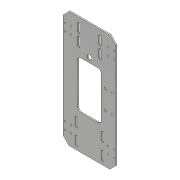
# Autodesk Inventor part: Plataina_eje_Y
Saved by Autodesk Inventor 2017 (Build 210142000, 142)
## iProperties
Created: 2018-02-17
Part Number: Plataina_eje_Y
Material: Aluminum 1100-O
Document SubType Name: Modeling
Designer: Juan Carlos Botero
Density: 2.7 g/cm^3
Appearance: Satin
Mass: 2621.1 g
Surface Area: 2107.17 cm^2
Volume: 970.778 cm^3
Author: Juan Carlos Botero
Autodesk Inventor part; units mm, degrees
ref_plane "YZ Plane" through (0, 0, 0) normal (1, 0, 0) x (0, 1, 0)
ref_plane "XZ Plane" through (0, 0, 0) normal (0, 1, 0) x (-1, 0, 0)
ref_plane "XY Plane" through (0, 0, 0) normal (0, 0, 1) x (1, 0, 0)
sketch "Sketch1" plane through (0, 0, 0) normal (0, 1, 0) x (-1, 0, 0)
  line L0 (111, 210) -> (-111, 210)
  line L1 (-111, 210) -> (-111, -210)
  line L2 (-111, -210) -> (111, -210)
  line L3 (111, -210) -> (111, 210)
  line L4 (111, 210) -> (-111, -210) construction
  line L5 (-111, 210) -> (111, -210) construction
  line L6 (111, -210) -> (75, -210) construction
  line L7 (75, -210) -> (75, -168) construction
  line L8 (75, -168) -> (111, -168) construction
  line L9 (111, -168) -> (111, -210) construction
  line L10 (-111, -210) -> (-75, -210) construction
  line L11 (-75, -210) -> (-75, -168) construction
  line L12 (-75, -168) -> (-111, -168) construction
  line L13 (-111, -168) -> (-111, -210) construction
  line L14 (-111, 210) -> (-75, 210) construction
  line L15 (-75, 210) -> (-75, 209.4774) construction
  line L16 (-75, 209.4774) -> (-111, 209.4774) construction
  line L17 (-111, 209.4774) -> (-111, 210) construction
  line L18 (111, 210) -> (75, 210) construction
  line L19 (75, 210) -> (75, 209.4774) construction
  line L20 (75, 209.4774) -> (111, 209.4774) construction
  line L21 (111, 209.4774) -> (111, 210) construction
  line L22 (75, -100) -> (-75, -100) construction
  line L23 (-75, -100) -> (-75, -210) construction
  line L24 (-75, -210) -> (75, -210) construction
  line L25 (75, -210) -> (75, -100) construction
  line L26 (75, -100) -> (-75, -210) construction
  line L27 (-75, -100) -> (75, -210) construction
  line L28 (37.5, 210) -> (-37.5, 210) construction
  line L29 (-37.5, 210) -> (-37.5, 60) construction
  line L30 (-37.5, 60) -> (37.5, 60) construction
  line L31 (37.5, 60) -> (37.5, 210) construction
  line L32 (37.5, 210) -> (-37.5, 60) construction
  line L33 (-37.5, 210) -> (37.5, 60) construction
  line L34 (-111, -210) -> (-111, -220)
  line L35 (-111, -220) -> (-86, -245)
  line L36 (-86, -245) -> (0, -245)
  line L37 (0, -245) -> (86, -245)
  line L38 (86, -245) -> (111, -220)
  line L39 (111, -220) -> (111, -210)
  line L40 (0, 0) -> (111, 0) construction
  line L41 (-111, 210) -> (111, 210)
  line L42 (-111, 210) -> (-111, 220)
  line L43 (-111, 220) -> (-86, 245)
  line L44 (-86, 245) -> (0, 245)
  line L45 (0, 245) -> (86, 245)
  line L46 (86, 245) -> (111, 220)
  line L47 (111, 220) -> (111, 210)
  point P0 (0, -155)
  point P1 (0, 135)
  point P2 (0, 210)
  dimension "d2" = 36
  dimension "d3" = 42
  dimension "d4" = 150
  dimension "d6" = 150
  dimension "d7" = 75
  dimension "d8" = 160
  dimension "d9" = 222
  dimension "d10" = 420
  dimension "d26" = 10
  dimension "d27" = 45
  dimension "d28" = 145
  dimension "d29" = 25
  dimension "d30" = 45
  constraints: 96 end point, 14 parallel, 9 midpoint, 9 perpendicular, 8 horizontal, 5 symmetric about line, 4 equal length, 3 point on line, 1 vertical
  measures "d2" distance of L7.end L8.end
  measures "d3" distance of L6.end L7.end
  measures "d4" distance of L6.end L10.end
  measures "d6" distance of L30.end L28.start
  measures "d7" distance of L28.start L28.end
  measures "d8" distance between parallel lines of L30 L22
  measures "d9" distance of L1.end L2.end
  measures "d10" distance of L0.end L1.end
  measures "d26" distance of L1.end L34.end
  measures "d27" angle of L10 L35
  measures "d28" distance between parallel lines of L22 L36
  measures "d29" distance from line of L35.end L34
  measures "d30" angle of L2 L38
extrude "Base" add sketch "Sketch1" along normal blind 5
sketch "Sketch2" plane through (0, 5, 0) normal (0, 1, 0) x (1, 0, 0)
  line L0 (111, -220) -> (111, 220) projected
  line L1 (-111, 220) -> (-111, -220) projected
  line L2 (-72, 159) -> (-108, 159)
  line L3 (-108, 159) -> (-108, 201)
  line L4 (-108, 201) -> (-72, 201)
  line L5 (-72, 201) -> (-72, 159)
  line L6 (-72, 159) -> (-108, 201) construction
  line L7 (-108, 159) -> (-72, 201) construction
  circle A0 centre (-103, 195.25) radius 2.55
  circle A1 centre (-77, 195.25) radius 2.55
  circle A2 centre (-77, 164.75) radius 2.55
  circle A3 centre (-103, 164.75) radius 2.55
  line L8 (-111, -220) -> (-86, -245) projected
  line L9 (-86, -245) -> (86, -245) projected
  line L10 (86, -245) -> (111, -220) projected
  line L11 (111, 220) -> (86, 245) projected
  line L12 (86, 245) -> (-86, 245) projected
  line L13 (-86, 245) -> (-111, 220) projected
  point P0 (0, 0)
  point P1 (-90, 180)
  dimension "d13" = 36
  dimension "d14" = 42
  dimension "d16" = 5
  dimension "d18" = 5.75
  dimension "d31" = 5.75
  dimension "d33" = 5
  dimension "d34" = 3
  dimension "d35" = 180
  dimension "d37" = 5.1
  constraints: 12 end point, 4 centre point, 3 equal radius, 2 horizontal alignment, 2 midpoint, 2 parallel, 2 vertical alignment, 1 horizontal, 1 perpendicular
  measures "d13" distance of L3.end L4.end
  measures "d14" distance of L3.end L2.end
  measures "d16" distance from line of L5 A1.centre
  measures "d18" distance from line of L2 A3.centre
  measures "d31" distance from line of L4 A0.centre
  measures "d33" distance from line of L3 A0.centre
  measures "d34" distance between parallel lines of L1 L3
  measures "d35" vertical distance of point (-90, 180) point (0, 0)
  measures "d37" diameter of A0
extrude "Rodamiento" cut sketch "Sketch2" against normal through all contours A0 | A1 | A2 | A3
mirror "Mirror1" about plane through (0, 0, 0) normal (1, 0, 0) of "Rodamiento"
mirror "Mirror2" about plane through (0, 0, 0) normal (0, 0, 1) of "Rodamiento", "Mirror1"
sketch "Sketch4" plane through (0, 5, 0) normal (0, 1, 0) x (1, 0, 0)
  line L0 (-55, 157.9056) -> (-55, 126.9056) construction
  line L1 (-60, 157.9056) -> (-60, 126.9056)
  line L2 (-50, 126.9056) -> (-50, 157.9056)
  arc A0 (-50, 157.9056) -> (-60, 157.9056) centre (-55, 157.9056) ccw
  arc A1 (-60, 126.9056) -> (-50, 126.9056) centre (-55, 126.9056) ccw
  line L3 (55, 157.9056) -> (55, 126.9056) construction
  line L4 (50, 157.9056) -> (50, 126.9056)
  line L5 (60, 126.9056) -> (60, 157.9056)
  arc A2 (60, 157.9056) -> (50, 157.9056) centre (55, 157.9056) ccw
  arc A3 (50, 126.9056) -> (60, 126.9056) centre (55, 126.9056) ccw
  line L6 (-55, 226.9056) -> (-55, 195.9056) construction
  line L7 (-60, 226.9056) -> (-60, 195.9056)
  line L8 (-50, 195.9056) -> (-50, 226.9056)
  arc A4 (-50, 226.9056) -> (-60, 226.9056) centre (-55, 226.9056) ccw
  arc A5 (-60, 195.9056) -> (-50, 195.9056) centre (-55, 195.9056) ccw
  line L9 (55, 226.9056) -> (55, 195.9056) construction
  line L10 (50, 226.9056) -> (50, 195.9056)
  line L11 (60, 195.9056) -> (60, 226.9056)
  arc A6 (60, 226.9056) -> (50, 226.9056) centre (55, 226.9056) ccw
  arc A7 (50, 195.9056) -> (60, 195.9056) centre (55, 195.9056) ccw
  line L12 (-55, 211.4056) -> (55, 211.4056) construction
  line L13 (86, 245) -> (-86, 245) construction
  point P0 (0, 0)
  point P1 (-55, 142.4056)
  point P2 (55, 142.4056)
  point P3 (0, 245)
  point P4 (0, 211.4056)
  dimension "d38" = 10
  dimension "d40" = 10
  dimension "d42" = 10
  dimension "d43" = 31
  dimension "d44" = 10
  dimension "d47" = 110
  dimension "d78" = 100
  constraints: 34 end point, 16 point on circle, 16 tangent, 8 centre point, 6 midpoint, 4 parallel, 4 vertical, 3 equal length, 3 vertical alignment, 2 horizontal alignment, 1 horizontal
  measures "d38" diameter of A1
  measures "d40" diameter of A3
  measures "d42" diameter of A5
  measures "d43" distance of L6.start L6.end
  measures "d44" diameter of A7
  measures "d47" distance of L12.start L12.end
  measures "d78" distance of L0.end L6.start
extrude "Extrusion4" cut sketch "Sketch4" against normal through all
sketch "Sketch6" plane through (0, 5, 0) normal (0, 1, 0) x (1, 0, 0)
  line L0 (50, 100) -> (-50, 100)
  line L1 (-50, 100) -> (-50, -100)
  line L2 (-50, -100) -> (50, -100)
  line L3 (50, -100) -> (50, 100)
  line L4 (50, 100) -> (-50, -100) construction
  line L5 (-50, 100) -> (50, -100) construction
  point P0 (0, 0)
  dimension "d55" = 100
  dimension "d56" = 200
  constraints: 12 end point, 2 midpoint, 2 parallel, 1 horizontal, 1 perpendicular
  measures "d55" distance of L1.end L2.end
  measures "d56" distance of L0.end L1.end
extrude "Extrusion6" cut sketch "Sketch6" against normal blind 20
sketch "Sketch10" plane through (0, 5, 0) normal (0, 1, 0) x (1, 0, 0)
  circle A0 centre (0, -120) radius 10
  line L0 (50, -100) -> (-50, -100) projected
  point P0 (0, 0)
  dimension "d71" = 20
  dimension "d77" = 20
  constraints: 1 centre point, 1 vertical alignment
  measures "d71" diameter of A0
  measures "d77" distance from line of L0 A0.centre
extrude "Extrusion10" cut sketch "Sketch10" against normal through all
fillet "Fillet1" radius 15 4 edges at (50, 2.5, -100) (-50, 2.5, -100) (-50, 2.5, 100) (50, 2.5, 100)
sketch "Sketch12" plane through (0, 5, 0) normal (0, 1, 0) x (1, 0, 0)
  line L0 (45, -190) -> (45, -220) construction
  line L1 (40, -190) -> (40, -220)
  line L2 (50, -220) -> (50, -190)
  arc A0 (50, -190) -> (40, -190) centre (45, -190) ccw
  arc A1 (40, -220) -> (50, -220) centre (45, -220) ccw
  line L3 (-45, -190) -> (-45, -220) construction
  line L4 (-50, -190) -> (-50, -220)
  line L5 (-40, -220) -> (-40, -190)
  arc A2 (-40, -190) -> (-50, -190) centre (-45, -190) ccw
  arc A3 (-50, -220) -> (-40, -220) centre (-45, -220) ccw
  line L6 (45, -205) -> (-45, -205) construction
  circle A4 centre (0, -120) radius 10 projected
  line L7 (-50, -85) -> (-50, 85) projected
  arc A5 (-35, 100) -> (-50, 85) centre (-35, 85) ccw projected
  line L8 (-35, 100) -> (35, 100) projected
  arc A6 (50, 85) -> (35, 100) centre (35, 85) ccw projected
  line L9 (50, 85) -> (50, -85) projected
  arc A7 (35, -100) -> (50, -85) centre (35, -85) ccw projected
  line L10 (35, -100) -> (-35, -100) projected
  arc A8 (-50, -85) -> (-35, -100) centre (-35, -85) ccw projected
  arc A9 (-60, 195.9056) -> (-50, 195.9056) centre (-55, 195.9056) ccw projected
  line L11 (-60, 195.9056) -> (-60, 226.9056) projected
  arc A10 (-50, 226.9056) -> (-60, 226.9056) centre (-55, 226.9056) ccw projected
  line L12 (-50, 226.9056) -> (-50, 195.9056) projected
  arc A11 (-60, 126.9056) -> (-50, 126.9056) centre (-55, 126.9056) ccw projected
  line L13 (-60, 126.9056) -> (-60, 157.9056) projected
  arc A12 (-50, 157.9056) -> (-60, 157.9056) centre (-55, 157.9056) ccw projected
  line L14 (-50, 157.9056) -> (-50, 126.9056) projected
  arc A13 (50, 126.9056) -> (60, 126.9056) centre (55, 126.9056) ccw projected
  line L15 (50, 126.9056) -> (50, 157.9056) projected
  arc A14 (60, 157.9056) -> (50, 157.9056) centre (55, 157.9056) ccw projected
  line L16 (60, 157.9056) -> (60, 126.9056) projected
  arc A15 (50, 195.9056) -> (60, 195.9056) centre (55, 195.9056) ccw projected
  line L17 (50, 195.9056) -> (50, 226.9056) projected
  arc A16 (60, 226.9056) -> (50, 226.9056) centre (55, 226.9056) ccw projected
  line L18 (60, 226.9056) -> (60, 195.9056) projected
  circle A17 centre (77, -164.75) radius 2.55 projected
  circle A18 centre (103, -164.75) radius 2.55 projected
  circle A19 centre (77, -195.25) radius 2.55 projected
  circle A20 centre (103, -195.25) radius 2.55 projected
  circle A21 centre (-77, -164.75) radius 2.55 projected
  circle A22 centre (-103, -164.75) radius 2.55 projected
  circle A23 centre (-77, -195.25) radius 2.55 projected
  circle A24 centre (-103, -195.25) radius 2.55 projected
  circle A25 centre (77, 164.75) radius 2.55 projected
  circle A26 centre (103, 164.75) radius 2.55 projected
  circle A27 centre (77, 195.25) radius 2.55 projected
  circle A28 centre (103, 195.25) radius 2.55 projected
  circle A29 centre (-77, 164.75) radius 2.55 projected
  circle A30 centre (-103, 195.25) radius 2.55 projected
  circle A31 centre (-77, 195.25) radius 2.55 projected
  circle A32 centre (-103, 164.75) radius 2.55 projected
  line L19 (-111, 220) -> (-111, -220) projected
  line L20 (-111, -220) -> (-86, -245) projected
  line L21 (-86, -245) -> (86, -245) projected
  line L22 (86, -245) -> (111, -220) projected
  line L23 (111, -220) -> (111, 220) projected
  line L24 (111, 220) -> (86, 245) projected
  line L25 (86, 245) -> (-86, 245) projected
  line L26 (-86, 245) -> (-111, 220) projected
  line L27 (103, -164.75) -> (77, -195.25) construction
  line L28 (45, -140) -> (45, -170) construction
  line L29 (40, -140) -> (40, -170)
  line L30 (50, -170) -> (50, -140)
  arc A33 (50, -140) -> (40, -140) centre (45, -140) ccw
  arc A34 (40, -170) -> (50, -170) centre (45, -170) ccw
  line L31 (-45, -140) -> (-45, -170) construction
  line L32 (-50, -140) -> (-50, -170)
  line L33 (-40, -170) -> (-40, -140)
  arc A35 (-40, -140) -> (-50, -140) centre (-45, -140) ccw
  arc A36 (-50, -170) -> (-40, -170) centre (-45, -170) ccw
  line L34 (45, -155) -> (-45, -155) construction
  line L35 (45, -140) -> (45, -220)
  point P0 (0, 0)
  point P1 (0, -205)
  point P2 (90, -180)
  point P3 (0, -155)
  point P4 (45, -180)
  dimension "d79" = 90
  dimension "d80" = 5
  dimension "d81" = 30
  dimension "d84" = 90
  dimension "d85" = 5
  dimension "d86" = 30
  dimension "d88" = 50
  constraints: 40 end point, 16 point on circle, 16 tangent, 8 centre point, 8 midpoint, 8 parallel, 2 equal radius, 2 horizontal, 2 vertical, 2 vertical alignment, 1 horizontal alignment
  measures "d79" distance of L6.start L6.end
  measures "d80" radius of A1
  measures "d81" distance of L0.start L0.end
  measures "d84" distance of L34.start L34.end
  measures "d85" radius of A34
  measures "d86" distance of L28.start L28.end
  measures "d88" distance of L28.start L0.start
extrude "Extrusion12" cut sketch "Sketch12" against normal through all contours A0 L2 A1 L1 | A34 L29 A33 L30 | A2 L5 A3 L4 | A35 L33 A36 L32
sketch "Sketch15" plane through (0, 5, 0) normal (0, 1, 0) x (1, 0, 0)
  circle A0 centre (97.4006, 40) radius 4.05
  circle A1 centre (67.4006, 40) radius 4.05
  circle A2 centre (97.4006, -40) radius 4.05
  circle A3 centre (67.4006, -40) radius 4.05
  line L0 (67.4006, 40) -> (97.4006, 40) construction
  line L1 (97.4006, 40) -> (97.4006, -40) construction
  line L2 (97.4006, -40) -> (67.4006, -40) construction
  line L3 (67.4006, -40) -> (67.4006, 40) construction
  line L4 (67.4006, 40) -> (97.4006, -40) construction
  line L5 (97.4006, 40) -> (67.4006, -40) construction
  point P0 (0, 0)
  point P1 (82.4006, 0)
  point P2 (82.4006, 0)
  dimension "d94" = 8.1
  dimension "d95" = 30
  dimension "d96" = 80
  constraints: 12 end point, 4 centre point, 3 coincident, 3 equal radius, 3 midpoint, 2 horizontal alignment, 2 parallel, 2 vertical alignment, 1 horizontal, 1 perpendicular
  measures "d94" diameter of A0
  measures "d95" distance of A1.centre A0.centre
  measures "d96" distance of L0.end L1.end
extrude "Extrusion14" cut sketch "Sketch15" against normal through all
sketch "Sketch13" plane through (0, 5, 0) normal (0, 1, 0) x (1, 0, 0)
  line L0 (95.5, 45) -> (65.5, 45) construction
  line L1 (95.5, 49) -> (65.5, 49)
  line L2 (65.5, 41) -> (95.5, 41)
  arc A0 (95.5, 41) -> (95.5, 49) centre (95.5, 45) ccw
  arc A1 (65.5, 49) -> (65.5, 41) centre (65.5, 45) ccw
  line L3 (95.5, -45) -> (65.5, -45) construction
  line L4 (95.5, -41) -> (65.5, -41)
  line L5 (65.5, -49) -> (95.5, -49)
  arc A2 (95.5, -49) -> (95.5, -41) centre (95.5, -45) ccw
  arc A3 (65.5, -41) -> (65.5, -49) centre (65.5, -45) ccw
  line L6 (80.5, 45) -> (80.5, -45) construction
  arc A4 (-40, -140) -> (-50, -140) centre (-45, -140) ccw projected
  line L7 (-40, -140) -> (-40, -170) projected
  arc A5 (-50, -170) -> (-40, -170) centre (-45, -170) ccw projected
  line L8 (-50, -170) -> (-50, -140) projected
  arc A6 (40, -220) -> (50, -220) centre (45, -220) ccw projected
  line L9 (40, -220) -> (40, -190) projected
  arc A7 (50, -190) -> (40, -190) centre (45, -190) ccw projected
  line L10 (50, -190) -> (50, -220) projected
  arc A8 (-50, -220) -> (-40, -220) centre (-45, -220) ccw projected
  line L11 (-50, -220) -> (-50, -190) projected
  arc A9 (-40, -190) -> (-50, -190) centre (-45, -190) ccw projected
  line L12 (-40, -190) -> (-40, -220) projected
  arc A10 (40, -170) -> (50, -170) centre (45, -170) ccw projected
  line L13 (40, -170) -> (40, -140) projected
  arc A11 (50, -140) -> (40, -140) centre (45, -140) ccw projected
  line L14 (50, -140) -> (50, -170) projected
  circle A12 centre (0, -120) radius 10 projected
  line L15 (-50, -85) -> (-50, 85) projected
  arc A13 (-35, 100) -> (-50, 85) centre (-35, 85) ccw projected
  line L16 (-35, 100) -> (35, 100) projected
  arc A14 (50, 85) -> (35, 100) centre (35, 85) ccw projected
  line L17 (50, 85) -> (50, -85) projected
  arc A15 (35, -100) -> (50, -85) centre (35, -85) ccw projected
  line L18 (35, -100) -> (-35, -100) projected
  arc A16 (-50, -85) -> (-35, -100) centre (-35, -85) ccw projected
  arc A17 (-60, 195.9056) -> (-50, 195.9056) centre (-55, 195.9056) ccw projected
  line L19 (-60, 195.9056) -> (-60, 226.9056) projected
  arc A18 (-50, 226.9056) -> (-60, 226.9056) centre (-55, 226.9056) ccw projected
  line L20 (-50, 226.9056) -> (-50, 195.9056) projected
  arc A19 (-60, 126.9056) -> (-50, 126.9056) centre (-55, 126.9056) ccw projected
  line L21 (-60, 126.9056) -> (-60, 157.9056) projected
  arc A20 (-50, 157.9056) -> (-60, 157.9056) centre (-55, 157.9056) ccw projected
  line L22 (-50, 157.9056) -> (-50, 126.9056) projected
  arc A21 (50, 126.9056) -> (60, 126.9056) centre (55, 126.9056) ccw projected
  line L23 (50, 126.9056) -> (50, 157.9056) projected
  arc A22 (60, 157.9056) -> (50, 157.9056) centre (55, 157.9056) ccw projected
  line L24 (60, 157.9056) -> (60, 126.9056) projected
  arc A23 (50, 195.9056) -> (60, 195.9056) centre (55, 195.9056) ccw projected
  line L25 (50, 195.9056) -> (50, 226.9056) projected
  arc A24 (60, 226.9056) -> (50, 226.9056) centre (55, 226.9056) ccw projected
  line L26 (60, 226.9056) -> (60, 195.9056) projected
  circle A25 centre (77, -164.75) radius 2.55 projected
  circle A26 centre (103, -164.75) radius 2.55 projected
  circle A27 centre (77, -195.25) radius 2.55 projected
  circle A28 centre (103, -195.25) radius 2.55 projected
  circle A29 centre (-77, -164.75) radius 2.55 projected
  circle A30 centre (-103, -164.75) radius 2.55 projected
  circle A31 centre (-77, -195.25) radius 2.55 projected
  circle A32 centre (-103, -195.25) radius 2.55 projected
  circle A33 centre (77, 164.75) radius 2.55 projected
  circle A34 centre (103, 164.75) radius 2.55 projected
  circle A35 centre (77, 195.25) radius 2.55 projected
  circle A36 centre (103, 195.25) radius 2.55 projected
  circle A37 centre (-77, 164.75) radius 2.55 projected
  circle A38 centre (-103, 195.25) radius 2.55 projected
  circle A39 centre (-77, 195.25) radius 2.55 projected
  circle A40 centre (-103, 164.75) radius 2.55 projected
  line L27 (-111, 220) -> (-111, -220) projected
  line L28 (-111, -220) -> (-86, -245) projected
  line L29 (-86, -245) -> (86, -245) projected
  line L30 (86, -245) -> (111, -220) projected
  line L31 (111, -220) -> (111, 220) projected
  line L32 (111, 220) -> (86, 245) projected
  line L33 (86, 245) -> (-86, 245) projected
  line L34 (-86, 245) -> (-111, 220) projected
  line L35 (111, 0) -> (50, 0) construction
  point P0 (0, 0)
  point P1 (80.5, 0)
  dimension "d89" = 90
  dimension "d90" = 30
  dimension "d91" = 4
  constraints: 20 end point, 8 point on circle, 8 tangent, 6 midpoint, 4 centre point, 4 parallel, 1 equal radius, 1 horizontal, 1 horizontal alignment, 1 vertical
  measures "d89" distance of L6.start L6.end
  measures "d90" distance of L3.start L3.end
  measures "d91" radius of A0
equation "\"d2\" = Rodamiento_d_a"
equation "\"d3\" = Rodamiento_d_b"
equation "\"d13\" = Rodamiento_d_a"
equation "\"d14\" = Rodamiento_d_b"
equation "\"d16\" = d15"
equation "\"d18\" = Rodamiento_d__tornillo_2"
equation "\"d31\" = d18"
equation "\"d33\" = Rodamiento_d_tornillo_1"
equation "\"d15\" = Rodamiento_d_tornillo_1"
equation "\"d17\" = Rodamiento_d_tornillo_1"
equation "\"Rodamiento_d_a\" = 36"
equation "\"Rodamiento_d_b\" = 42"
equation "\"Rodamiento_d_tornillo_1\" = 5"
equation "\"Rodamiento_d__tornillo_2\" = 5.75"
